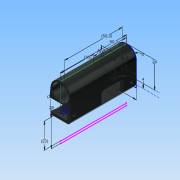
# Autodesk Inventor part: лЕВАЯ  КАРЕТКА  Y
Saved by Autodesk Inventor 2017 (Build 210142000, 142)
## iProperties
Part Number: лЕВАЯ  КАРЕТКА  Y
Material: Типовые
Document SubType Name: Modeling
Designer: Max
Mass: 9.94822 g
Surface Area: 102.595 cm^2
Volume: 9.94822 cm^3
Density: 1 g/cm^3
Appearance: Оружейный металл — полированный
Author: Max
Autodesk Inventor part; units mm, degrees
ref_plane "YZ Plane" through (0, 0, 0) normal (1, 0, 0) x (0, 1, 0)
ref_plane "XZ Plane" through (0, 0, 0) normal (0, 1, 0) x (-1, 0, 0)
ref_plane "XY Plane" through (0, 0, 0) normal (0, 0, 1) x (1, 0, 0)
sketch "Эскиз1" plane through (0, 0, 0) normal (0, 1, 0) x (-1, 0, 0)
  circle A0 centre (0, 0) radius 7.5
  line L0 (-9, 0) -> (-9, -21.5)
  line L1 (9.9923, -7.3759) -> (8.9305, 1.1166)
  arc A1 (8.9305, 1.1166) -> (-9, 0) centre (0, 0) ccw
  line L2 (-30.7605, -15) -> (-1.3474, -15) construction
  line L3 (-30.2885, -19) -> (-1.3474, -19) construction
  line L4 (-6, -8.5) -> (9, -8.5)
  arc A2 (9, -8.5) -> (9.9923, -7.3759) centre (9, -7.5) ccw
  circle A3 centre (0, 0) radius 4 construction
  line L5 (-9, -21.5) -> (8.7, -21.5)
  line L6 (8.7, -21.5) -> (8.7, -19.15)
  line L7 (-6, -19.15) -> (-6, -8.5)
  line L8 (-6, -19.15) -> (8.7, -19.15)
  dimension "d0" = 15
  dimension "d13" = 9
  dimension "d94" = 24
  dimension "d95" = 4
  dimension "d98" = 1
  dimension "d101" = 8
  dimension "d103" = 4.5
  dimension "d105" = 17.5
  dimension "d106" = 2.35
  dimension "d107" = 3
  dimension "d108" = 19
  dimension "d109" = 17.7
  constraints: 18 end point, 4 centre point, 4 horizontal, 4 point on circle, 4 tangent, 3 coincident, 2 perpendicular, 1 vertical
  measures "d0" diameter of A0
  measures "d13" radius of A1
  measures "d95" distance between parallel lines of L3 L2
  measures "d98" radius of A2
  measures "d101" diameter of A3
  measures "d103" distance edge to line of A3 L4
  measures "d105" distance edge to line of A3 L5
  measures "d106" distance between parallel lines of L5 L8
  measures "d107" distance between parallel lines of L0 L7
  measures "d109" distance between parallel lines of L6 L0
extrude "Выдавливание1" add sketch "Эскиз1" against normal blind 60
sketch "Эскиз5" plane through (0, 0, 0) normal (1, 0, 0) x (0, 1, 0)
  line L0 (-3.85, -15) -> (-56.15, -15) construction
  circle A0 centre (-56.15, -15) radius 1.5
  circle A1 centre (-3.85, -15) radius 1.5
  circle A2 centre (-3.85, -15) radius 3
  circle A3 centre (-56.15, -15) radius 3
  line L1 (0, 9) -> (-60, 9) projected
  line L2 (-60, -40) -> (0, -40) projected
  line L3 (0, -38) -> (-60, -38) projected
  line L4 (-30, 9) -> (-30, -12)
  line L5 (-60, -7.5) -> (-60, 7.5) projected
  line L6 (0, 7.5) -> (0, -7.5) projected
  circle A4 centre (-3.85, -15) radius 4 construction
  circle A5 centre (-56.15, -15) radius 4 construction
  point P0 (0, 0)
  dimension "d62" = 3
  dimension "d63" = 3
  dimension "d64" = 6
  dimension "d65" = 6
  dimension "d66" = 28
  dimension "d67" = 24
  dimension "d68" = 23
  dimension "d69" = 30
  dimension "d70" = 30
  dimension "d71" = 8
  dimension "d79" = 8
  dimension "d80" = 60.3
  dimension "d81" = 52.3
  constraints: 6 centre point, 6 coincident, 4 end point, 1 horizontal, 1 midpoint, 1 symmetric about line, 1 vertical
  measures "d62" diameter of A0
  measures "d63" diameter of A1
  measures "d64" diameter of A2
  measures "d65" diameter of A3
  measures "d67" distance from line of L1 L0.end
  measures "d68" distance from line of L0.end L3
  measures "d69" distance between parallel lines of L4 L5
  measures "d70" distance between parallel lines of L4 L6
  measures "d71" diameter of A4
  measures "d79" diameter of A5
  measures "d81" distance of L0.start L0.end
extrude "Выдавливание8" cut sketch "Эскиз5" along normal blind 25 contours A0 | A1
fillet "Сопряжение5" radius 3 1 edges at (9, -30, -21.5)
fillet "Сопряжение6" radius 1 1 edges at (6, -30, -19.15)
sketch "Эскиз7" plane through (6, -60, -8.5) normal (-1, 0, 0) x (0, 0, 1)
  line L0 (0, 60) -> (0, 0) projected
  line L1 (-2, 48.3) -> (-8.65, 48.3)
  line L2 (-10.65, 46.3) -> (-10.65, 30.3)
  line L3 (-8.65, 28.3) -> (-2, 28.3)
  line L4 (0, 30.3) -> (0, 46.3)
  arc A0 (0, 46.3) -> (-2, 48.3) centre (-2, 46.3) ccw
  arc A1 (-8.65, 48.3) -> (-10.65, 46.3) centre (-8.65, 46.3) ccw
  arc A2 (-10.65, 30.3) -> (-8.65, 28.3) centre (-8.65, 30.3) ccw
  arc A3 (-2, 28.3) -> (0, 30.3) centre (-2, 30.3) ccw
  line L5 (-13, 60) -> (-13, 0) projected
  line L6 (-9.65, 60) -> (0, 60) projected
  point P0 (8.5, 60)
  point P1 (0, 48.3)
  point P2 (-10.65, 28.3)
  dimension "d112" = 2
  dimension "d114" = 2.35
  dimension "d115" = 11.7
  dimension "d116" = 20
  constraints: 8 end point, 8 point on circle, 8 tangent, 5 point on line, 4 centre point, 3 equal radius, 2 parallel, 1 horizontal, 1 perpendicular
  measures "d112" radius of A0
  measures "d114" distance between parallel lines of L5 L2
  measures "d115" distance between parallel lines of L6 L1
  measures "d116" distance between parallel lines of L3 L1
extrude "Выдавливание11" cut sketch "Эскиз7" along normal mid plane 30
sketch "Эскиз8" plane through (-8.7, 0, -21.5) normal (-1, 0, 0) x (0, 0, 1)
  line L0 (0, 0) -> (2.35, 0) projected
  line L1 (0, 0) -> (0, -60) projected
  line L2 (2.35, -60) -> (0, -60) projected
  line L3 (2.35, 0) -> (2.35, -60) projected
  line L4 (2.35, -2.6) -> (0, -2.6)
  line L5 (0, 0) -> (0, -60) projected
  line L6 (2.35, 0) -> (2.35, -13.7) projected
  line L7 (2.35, -6.1) -> (0, -6.1)
  line L8 (2.35, 0) -> (2.35, -60) projected
  line L9 (2.35, -39.9) -> (0, -39.9)
  line L10 (2.35, -41.4) -> (0, -41.4)
  line L11 (2.35, -39.9) -> (0, -39.9)
  line L12 (0, -39.9) -> (0, -41.4)
  line L13 (0, -41.4) -> (2.35, -41.4)
  line L14 (2.35, -41.4) -> (2.35, -39.9)
  line L15 (2.35, -2.6) -> (0, -2.6)
  line L16 (0, -2.6) -> (0, -6.1)
  line L17 (0, -6.1) -> (2.35, -6.1)
  line L18 (2.35, -6.1) -> (2.35, -2.6)
  line L19 (0, -6.1) -> (2.35, -6.1)
  line L20 (2.35, -6.1) -> (2.35, -10.1)
  line L21 (2.35, -10.1) -> (0, -10.1)
  line L22 (0, -10.1) -> (0, -6.1)
  point P0 (21.5, 0)
  dimension "d119" = 18.6
  dimension "d120" = 1.5
  dimension "d121" = 2.6
  dimension "d122" = 3.5
  dimension "d125" = 4
  constraints: 32 end point, 9 point on line, 7 parallel, 5 perpendicular, 4 horizontal
  measures "d119" distance between parallel lines of L2 L10
  measures "d120" distance between parallel lines of L10 L9
  measures "d121" distance between parallel lines of L0 L15
  measures "d122" distance between parallel lines of L7 L4
  measures "d125" distance between parallel lines of L19 L21
extrude "Выдавливание12" cut sketch "Эскиз8" against normal blind 7 contours L7 L3 L21 L1 | L9 L3 L10 L1
extrude "Выдавливание13" cut sketch "Эскиз8" against normal blind 11 contours L0 L3 L4 L1
fillet "Сопряжение7" radius 3 2 edges at (6, -6.85, -8.5) (6, -44.85, -8.5)
chamfer "Фаска1" distance 3 angle 45 3 edges at (-8.7, -10.1, -20.325) (-8.7, -39.9, -20.325) (-8.7, -41.4, -20.325)
sketch "Эскиз9" plane through (6, -60, -21.5) normal (0, 0, -1) x (-1, 0, 0)
  circle A0 centre (11.3923, 38.75) radius 1.5
  line L0 (3, 60) -> (15, 60) projected
  line L1 (15.9923, 60) -> (15.9923, 0) projected
  point P0 (6, 60)
  dimension "d132" = 3
  dimension "d133" = 21.25
  dimension "d134" = 4.6
  constraints: 1 centre point
  measures "d132" diameter of A0
  measures "d133" distance from line of L0 A0.centre
  measures "d134" distance from line of L1 A0.centre
extrude "Выдавливание14" cut sketch "Эскиз9" against normal blind 21
sketch "Эскиз10" plane through (0, 0, 0) normal (1, 0, 0) x (0, 1, 0)
  line L0 (0, 7.5) -> (0, -7.5) projected
  line L1 (0, -5.0093) -> (-56.3609, -5.0093)
  circle A0 centre (-13, -5.0093) radius 1.5
  circle A1 centre (-47, -5.0093) radius 1.5
  line L2 (-60, 1.1166) -> (-60, -7.3759) projected
  point P0 (0, 0)
  dimension "d137" = 3
  dimension "d138" = 3
  dimension "d139" = 34
  dimension "d146" = 13
  dimension "d147" = 13
  constraints: 3 point on line, 2 centre point, 2 end point, 1 horizontal
  measures "d137" diameter of A0
  measures "d138" diameter of A1
  measures "d139" distance of A1.centre A0.centre
  measures "d146" distance from line of L0 A0.centre
  measures "d147" distance from line of L2 A1.centre
extrude "Выдавливание15" cut sketch "Эскиз10" against normal blind 10
thread "Резьба1" size "M3x0.5" class "6H" standard "ANSI Metric M Profile" full length
thread "Резьба2" size "M3x0.5" class "6H" standard "ANSI Metric M Profile" full length
sketch "Эскиз12" plane through (-9.8839, -47, -5.0093) normal (0, 1, 0) x (0, 0, 1)
  line L0 (1.5, 0) -> (1.5, 6.1586)
  line L1 (1.5, 6.1586) -> (1.1293, 6.1586)
  line L2 (1.1293, 6.1586) -> (1.1293, 0)
  line L3 (1.1293, 0) -> (1.5, 0)
  line L4 (0, -4.4314) -> (0, 22.7714) projected
  constraints: 8 end point
revolve "Вращение1" add sketch "Эскиз12" angle 360 about axis through (-9.8839, -47, -5.0093) along (1, 0, 0) separate body
sketch "Эскиз11" plane through (-9.8839, -47, -3.5093) normal (0, -1, 0) x (1, 0, 0)
  line L0 (-0.2918, -0.0255) -> (-0.2501, -0.0255) construction
  line L1 (0.0416, -0.3456) -> (-0.0001, -0.4257) construction
  line L2 (-0.5001, -0.4257) -> (-0.5418, -0.3456) construction
  line L3 (-0.2084, -0.0255) -> (-0.2501, 0.0546) construction
  line L4 (-0.2501, 0.0546) -> (-0.2918, -0.0255) construction
  line L5 (-0.5001, -0.4257) -> (-0.4584, -0.3456) construction
  line L6 (-0.2084, -0.0255) -> (-0.0418, -0.3456)
  line L7 (-0.5418, -0.3456) -> (-0.4584, -0.3456) construction
  arc A0 (-0.5418, -0.3456) -> (-0.5001, -0.3709) centre (-0.5001, -0.3239) ccw construction
  line L8 (0.0416, -0.3456) -> (-0.0418, -0.3456) construction
  line L9 (-0.5001, -0.4257) -> (-0.5001, -0.3456) construction
  line L10 (-0.0001, -0.4257) -> (-0.0001, -0.3456) construction
  line L11 (-0.2501, 0.0546) -> (-0.2501, -0.0002) construction
  line L12 (-0.5001, -0.3709) -> (-0.0001, -0.3709)
  arc A1 (-0.5001, -0.3709) -> (-0.4584, -0.3456) centre (-0.5001, -0.3239) ccw
  line L13 (-0.0418, -0.3456) -> (-0.0001, -0.4257) construction
  line L14 (-0.4584, -0.3456) -> (-0.2918, -0.0255)
  line L15 (-0.0001, -0.0002) -> (-0.0001, 0.0177)
  line L16 (-0.0001, 0.0177) -> (-0.0001, -0.0002)
  line L17 (-0.0001, -0.0002) -> (0.0334, -0.0002)
  arc A2 (-0.0418, -0.3456) -> (-0.0001, -0.3709) centre (-0.0001, -0.3239) ccw
  arc A3 (-0.0001, -0.3709) -> (0.0416, -0.3456) centre (-0.0001, -0.3239) ccw construction
  arc A4 (-0.2501, -0.0002) -> (-0.2918, -0.0255) centre (-0.2501, -0.0471) ccw
  arc A5 (-0.2084, -0.0255) -> (-0.2501, -0.0002) centre (-0.2501, -0.0471) ccw
  line L18 (-0.2501, -0.0002) -> (-0.2501, -0.0255) construction
  line L19 (-0.2501, -0.0255) -> (-0.2084, -0.0255) construction
  dimension "d148" = 55
  dimension "d149" = 0.08
  dimension "d150" = 0.08
  dimension "Эскиз11_ThreadOffset" = 0
  dimension "Эскиз11_MajorRadius" = 0.3707
  dimension "d153" = 0.5
  dimension "Эскиз11_MinorRadius" = 0
  constraints: 40 end point, 12 point on circle, 10 parallel, 8 tangent, 6 centre point, 6 collinear, 2 midpoint, 2 point on line, 1 horizontal, 1 perpendicular, 3 other
  measures "d148" angle of L6 L14
  measures "d149" distance of L3.end L0.end
  measures "d150" distance of L1.end L10.end
  measures "Эскиз11_ThreadOffset" distance between parallel lines of L15 L10
  measures "Эскиз11_MajorRadius" distance from line of L12 L15.start
  measures "d153" distance from line of L1.end L9
  measures "Эскиз11_MinorRadius" distance edge to line of A5 L17
coil "Пружина1" sketch "Эскиз11" operation cut axis through (-9.8839, -47, -5.0093) along (1, 0, 0) pitch 0.5005 turns 14.302812 hand right bodies 2
sketch "Эскиз14" plane through (-9.8839, -13, -5.0093) normal (0, 1, 0) x (0, 0, 1)
  line L0 (1.5, 0) -> (1.5, 6.1586)
  line L1 (1.5, 6.1586) -> (1.1293, 6.1586)
  line L2 (1.1293, 6.1586) -> (1.1293, 0)
  line L3 (1.1293, 0) -> (1.5, 0)
  line L4 (0, -4.4314) -> (0, 22.7714) projected
  constraints: 8 end point
revolve "Вращение2" add sketch "Эскиз14" angle 360 about axis through (-9.8839, -13, -5.0093) along (1, 0, 0) separate body
sketch "Эскиз13" plane through (-9.8839, -13, -3.5093) normal (0, -1, 0) x (1, 0, 0)
  line L0 (-0.2918, -0.0255) -> (-0.2501, -0.0255) construction
  line L1 (0.0416, -0.3456) -> (-0.0001, -0.4257) construction
  line L2 (-0.5001, -0.4257) -> (-0.5418, -0.3456) construction
  line L3 (-0.2084, -0.0255) -> (-0.2501, 0.0546) construction
  line L4 (-0.2501, 0.0546) -> (-0.2918, -0.0255) construction
  line L5 (-0.5001, -0.4257) -> (-0.4584, -0.3456) construction
  line L6 (-0.2084, -0.0255) -> (-0.0418, -0.3456)
  line L7 (-0.5418, -0.3456) -> (-0.4584, -0.3456) construction
  arc A0 (-0.5418, -0.3456) -> (-0.5001, -0.3709) centre (-0.5001, -0.3239) ccw construction
  line L8 (0.0416, -0.3456) -> (-0.0418, -0.3456) construction
  line L9 (-0.5001, -0.4257) -> (-0.5001, -0.3456) construction
  line L10 (-0.0001, -0.4257) -> (-0.0001, -0.3456) construction
  line L11 (-0.2501, 0.0546) -> (-0.2501, -0.0002) construction
  line L12 (-0.5001, -0.3709) -> (-0.0001, -0.3709)
  arc A1 (-0.5001, -0.3709) -> (-0.4584, -0.3456) centre (-0.5001, -0.3239) ccw
  line L13 (-0.0418, -0.3456) -> (-0.0001, -0.4257) construction
  line L14 (-0.4584, -0.3456) -> (-0.2918, -0.0255)
  line L15 (-0.0001, -0.0002) -> (-0.0001, 0.0177)
  line L16 (-0.0001, 0.0177) -> (-0.0001, -0.0002)
  line L17 (-0.0001, -0.0002) -> (0.0334, -0.0002)
  arc A2 (-0.0418, -0.3456) -> (-0.0001, -0.3709) centre (-0.0001, -0.3239) ccw
  arc A3 (-0.0001, -0.3709) -> (0.0416, -0.3456) centre (-0.0001, -0.3239) ccw construction
  arc A4 (-0.2501, -0.0002) -> (-0.2918, -0.0255) centre (-0.2501, -0.0471) ccw
  arc A5 (-0.2084, -0.0255) -> (-0.2501, -0.0002) centre (-0.2501, -0.0471) ccw
  line L18 (-0.2501, -0.0002) -> (-0.2501, -0.0255) construction
  line L19 (-0.2501, -0.0255) -> (-0.2084, -0.0255) construction
  dimension "d166" = 55
  dimension "d167" = 0.08
  dimension "d168" = 0.08
  dimension "Эскиз13_ThreadOffset" = 0
  dimension "Эскиз13_MajorRadius" = 0.3707
  dimension "d171" = 0.5
  dimension "Эскиз13_MinorRadius" = 0
  constraints: 40 end point, 12 point on circle, 10 parallel, 8 tangent, 6 centre point, 6 collinear, 2 midpoint, 2 point on line, 1 horizontal, 1 perpendicular, 3 other
  measures "d166" angle of L6 L14
  measures "d167" distance of L3.end L0.end
  measures "d168" distance of L1.end L10.end
  measures "Эскиз13_ThreadOffset" distance between parallel lines of L15 L10
  measures "Эскиз13_MajorRadius" distance from line of L12 L15.start
  measures "d171" distance from line of L1.end L9
  measures "Эскиз13_MinorRadius" distance edge to line of A5 L17
coil "Пружина2" sketch "Эскиз13" operation cut axis through (-9.8839, -13, -5.0093) along (1, 0, 0) pitch 0.5005 turns 14.302812 hand right bodies 3
equation "\"d148\" = d155"
equation "\"d149\" = 0.160083 * Эскиз11_Pitch"
equation "\"d150\" = 0.160083 * Эскиз11_Pitch"
equation "\"d153\" = Эскиз11_Pitch"
equation "\"d166\" = d173"
equation "\"d167\" = 0.160083 * Эскиз13_Pitch"
equation "\"d168\" = 0.160083 * Эскиз13_Pitch"
equation "\"d171\" = Эскиз13_Pitch"
equation "\"d155\" = 55deg"
equation "\"Эскиз11_Pitch\" = 0.5"
equation "\"d173\" = 55deg"
equation "\"Эскиз13_Pitch\" = 0.5"
